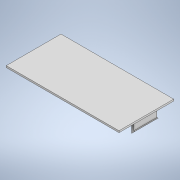
# Autodesk Inventor part: TapaOnixium
Saved by Autodesk Inventor 2021 (Build 250183000, 183)
## iProperties
Created: 2021-10-29
Part Number: TapaOnixium
Material: Genérico
Document SubType Name: Chapa
Designer: Juan Camilo
Density: 1 g/cm^3
Sheet Metal Rule: Por defecto_mm
Appearance: Valor por defecto
Author: Juan Camilo
Autodesk Inventor part; units mm, degrees
ref_plane "YZ Plane" through (0, 0, 0) normal (1, 0, 0) x (0, 1, 0)
ref_plane "XZ Plane" through (0, 0, 0) normal (0, 1, 0) x (-1, 0, 0)
ref_plane "XY Plane" through (0, 0, 0) normal (0, 0, 1) x (1, 0, 0)
sketch "Boceto1" plane through (0, 0, 0) normal (0, 1, 0) x (-1, 0, 0)
  line L0 (-15, 66) -> (-49, 66)
  line L1 (45, 18.438) -> (49, 18.438)
  line L2 (-49, 66) -> (49, 66)
  line L3 (49, 66) -> (49, 18.438)
  line L4 (49, 18.438) -> (-49, 18.438)
  line L5 (-49, 18.438) -> (-49, 66)
  line L6 (-47, 51) -> (-45, 51)
  line L7 (-47, 51) -> (-45, 51)
  line L8 (-45, 51) -> (-45, 31)
  line L9 (-45, 31) -> (-47, 31)
  line L10 (-47, 31) -> (-47, 51)
  line L11 (45, 51.5) -> (45, 42.5)
  line L12 (47, 51) -> (47, 31)
  line L13 (45, 51.5) -> (47, 51.5)
  line L14 (47, 51.5) -> (47, 31)
  line L15 (47, 31) -> (45, 31)
  line L16 (45, 31) -> (45, 51.5)
  point P0 (0, 0)
  constraints: 32 end point, 5 parallel, 3 horizontal, 3 perpendicular, 1 vertical, 3 other
extrude "Extrusión1" add sketch "Boceto1" along normal blind 1.5 contours L2 L3 L1 L4 L5 L0 | L6 L8 L9 L10 | L13 L14 L12 L15 L16 L11
sketch "Boceto2" plane through (0, 0, 0) normal (0, -1, 0) x (1, 0, 0)
  line L0 (-47, 51) -> (-45, 51)
  line L1 (-45, 51) -> (-45, 30.9876)
  line L2 (-45, 30.9876) -> (-47, 30.9876)
  line L3 (-47, 30.9876) -> (-47, 51)
  line L4 (45, 51) -> (47, 51)
  line L5 (47, 51) -> (47, 31)
  line L6 (47, 31) -> (45, 31)
  line L7 (45, 31) -> (45, 51)
  point P0 (0, 0)
  constraints: 16 end point, 4 parallel, 2 horizontal, 2 perpendicular
extrude "Extrusión2" add sketch "Boceto2" along normal blind 10
sketch "Boceto3" plane through (-47, 0, 30.9876) normal (-1, 0, 0) x (0, 0, 1)
  line L0 (0, -10) -> (20.0124, -10) projected
  line L1 (20.0124, 0) -> (20.0124, -10) projected
  line L2 (0, -10) -> (20.0124, -10)
  line L3 (20.0124, -10) -> (20.0124, -7)
  line L4 (20.0124, -7) -> (0, -7)
  line L5 (0, -7) -> (0, -10)
  dimension "d4" = 3
  constraints: 8 end point, 2 parallel, 1 horizontal, 1 perpendicular, 1 point on line
  measures "d4" distance of L4.end L0.start
extrude "Extrusión3" add sketch "Boceto3" along normal blind 1
sketch "Boceto5" plane through (47, 0, 51) normal (1, 0, 0) x (0, 0, -1)
  line L0 (20.0124, -10) -> (0, -10) projected
  line L1 (0, -10) -> (20.0124, -10)
  line L2 (20.0124, -10) -> (20.0124, -7)
  line L3 (20.0124, -7) -> (0, -7)
  line L4 (0, -7) -> (0, -10)
  point P0 (51, 0)
  dimension "d8" = 3
  constraints: 8 end point, 2 parallel, 1 horizontal, 1 perpendicular
  measures "d8" distance of L1.end L2.end
extrude "Extrusión4" add sketch "Boceto5" along normal blind 1
sketch "Boceto7" plane through (-49, 0, 66) normal (0, 0, 1) x (1, 0, 0)
  line L0 (49, 0) -> (49, 1.3987)
  line L1 (4, -10) -> (1, -10) projected
  line L2 (2, -7) -> (1, -7) projected
  line L3 (4, -10) -> (1, -10)
  line L4 (1, -10) -> (1, -7)
  line L5 (4, -7) -> (4, -10)
  line L6 (1, -7) -> (4, -10)
  line L7 (1, -10) -> (4, -10)
  line L8 (1, -7) -> (1, -10)
  line L9 (94, -10) -> (97, -10)
  line L10 (97, -10) -> (97, -7)
  line L11 (97, -7) -> (94, -10)
  constraints: 20 end point, 4 symmetric about line, 3 equal length, 1 horizontal, 1 perpendicular, 1 vertical
extrude "Extrusión5" cut sketch "Boceto7" against normal blind 48.25
equation "\"Radio_pliegue\" = Grosor"
equation "\"Anchura_desahogo_plegado\" = Grosor"
equation "\"Profundidad_desahogo_plegado\" = 0.5 * Grosor"
equation "\"Tamaño_destalonado\" = 4 * Grosor"
equation "\"Remanente_mínimo\" = 2 * Grosor"
equation "\"Radiodetransición\" = Radio_pliegue"
equation "\"Tamaño_de_radio_de_Jacobi\" = Radio_pliegue"
equation "\"TamañoSeparación\" = Grosor"
equation "\"Grosor\" = 0.5"
